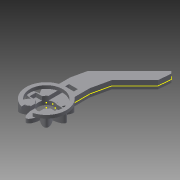
# Autodesk Inventor part: BrazoPinza2
Saved by Autodesk Inventor 2014 SP1 (Build 180222100, 222)
## iProperties
Created: 2013-11-10
Part Number: BrazoPinza2
Material: Genérico
Document SubType Name: Modeling
Designer: Gregorio
Density: 1 g/cm^3
Appearance: Valor por defecto
Author: Gregorio
Autodesk Inventor part; units mm, degrees
ref_plane "YZ Plane" through (0, 0, 0) normal (1, 0, 0) x (0, 1, 0)
ref_plane "XZ Plane" through (0, 0, 0) normal (0, 1, 0) x (-1, 0, 0)
ref_plane "XY Plane" through (0, 0, 0) normal (0, 0, 1) x (1, 0, 0)
sketch "Boceto1" plane through (0, 0, 0) normal (0, 0, 1) x (1, 0, 0)
  circle A0 centre (0, 0) radius 12.5
  circle A1 centre (0, 0) radius 4
  ellipse E0 centre (0, 4) end of major axis (0, 12.5) minor radius 3
  ellipse E1 centre (2.85, 2.8067) end of major axis (8.9175, 8.7595) minor radius 3
  ellipse E2 centre (4, 0) end of major axis (12.5, 0) minor radius 3
  ellipse E3 centre (2.85, -2.8067) end of major axis (8.8031, -8.8744) minor radius 3
  ellipse E4 centre (0, -4) end of major axis (0, -12.5) minor radius 3
  ellipse E5 centre (-2.85, -2.8067) end of major axis (-8.9175, -8.7595) minor radius 3
  ellipse E6 centre (-4, 0) end of major axis (-12.5, 0) minor radius 3
  ellipse E7 centre (-2.85, 2.8067) end of major axis (-8.8031, 8.8744) minor radius 3
  dimension "d1" = 8
  dimension "d4" = 3
  dimension "d5" = 3
  dimension "d6" = 3
  dimension "d7" = 3
  dimension "d8" = 3
  dimension "d9" = 3
  dimension "d10" = 3
  dimension "d11" = 3
  dimension "d0" = 25
  dimension "d12" = 2.85
  dimension "d14" = 2.85
  dimension "d15" = 2.85
  dimension "d16" = 2.85
  constraints: 2 coincident, 2 horizontal alignment, 2 vertical alignment, 1 centre point, 34 other
  measures "d0" diameter of A0
  measures "d12" horizontal distance of point (2.85, 2.807) point (0, 4)
  measures "d14" horizontal distance of point (-2.85, 2.807) point (0, 4)
  measures "d15" horizontal distance of point (0, -4) point (-2.85, -2.807)
  measures "d16" horizontal distance of point (2.85, -2.807) point (0, -4)
extrude "Extrusión1" add sketch "Boceto1" along normal blind 2 contours E2 E3 E6 E1 | E1 E2 E5 E0 | E3 E4 E7 E2 | E1 E6 A1 E5 E2 | E2 E7 A1 E6 E3 | E0 E1 E4 E7 | E0 E5 A1 E4 E1 | E4 E5 E0 E3 | E3 E0 A1 E7 E4 | E6 E3 E1 | E1 E3 A1 E6 | E5 A1 E0 E2 | E2 E0 E5 | E7 E4 E2 | E2 E4 A1 E7 | E6 A1 E1 E3 | E7 E0 E3 E6 | E7 E4 A1 E3 E0 | E0 E2 A1 E5 | E4 A1 E7 E1 | E1 E7 E4 | E5 E6 E1 E4 | E4 E1 A1 E0 E5 | E3 E5 A1 E0 | E0 E5 E3 | E7 A1 E2 E4 | E1 A1 E3 | E6 E5 A1 | A1 E3 E5 E6 | E0 A1 E2 | E5 E6 E0 A1 | E2 A1 E4 | E7 E6 A1 | A1 E4 E6 E7 | E6 E7 E1 A1 | E6 E7 E2 E5 | E6 E3 A1 E2 E7 | E3 A1 E6 E0 | E0 E6 E3 | E7 E1 A1 E4 | E5 E4 A1 | A1 E2 E4 E5 | E7 A1 E1 | E4 E5 E7 A1 | E5 E2 A1 E1 E6 | E4 E6 A1 E1 | E1 E6 E4 | E0 A1 E3 E5 | E0 E7 A1 | A1 E5 E7 E0 | E3 A1 E5 | E7 E0 E2 A1 | E1 E7 E5 E3 A1 | E5 E3 E0 E6 | E0 E6 E4 E2 A1 | E2 E0 E6 E4 A1 | E6 E4 E1 E7 | E6 E0 A1 E3 | E7 E5 E2 | E2 A1 E5 E7 | E6 A1 E0 | E3 E4 E6 A1 | A1 E4 E3 | A1 E1 E3 E4 | E4 E2 E7 E5 | A1 E7 E5 E3 E1 | E5 E7 A1 E2 | E1 A1 E4 E6 | E1 E0 A1 | A1 E6 E0 E1 | E4 A1 E6 | E0 E1 E3 A1 | A1 E3 E1 E7 E5 | E7 E5 E2 E0 | E1 E4 E5 E7 | E5 E7 E0 E3 | E0 E3 E4 E6 | E4 E6 E7 E2 | E2 E5 E6 E0 | E6 E0 E1 E4 | E3 E2 A1 | A1 E0 E2 E3 | E2 E3 E5 A1 | E5 A1 E7 | A1 E6 E4 E2 E0 | E3 E1 E6 E4 | E7 E2 E3 E5 | E3 E5 E6 E1 | E2 E1 A1 | A1 E7 E1 E2 | E1 E2 E4 A1 | A1 E4 E2 E0 E6 | E0 E6 E3 E1 | E7 E1 E2 E5 | E3 E6 E7 E1 | E1 E0 E5 E4 | E5 E4 E0 E7 | E0 E7 E4 E3 | E4 E3 E7 E6 | E7 E6 E3 E2 | E6 E5 E1 E0 | E2 E1 E6 E5 | E2 E0 E5 E3 | E5 E3 E1 E7 A1 | E2 E4 E5 E0 | E6 E1 E2 E4 | E3 E2 E6 E5 | E6 E5 E2 E1 | E1 E7 E4 E2 | E0 E2 E3 E6 | E4 E7 E0 E2 | E7 E6 E2 E1 | E3 E2 E7 E6 | E1 E5 E0 | E5 E0 E4 | E0 E4 E7 | E4 E7 E3 | E7 E3 E6 | E3 E6 E2 | E6 E1 E5 | E2 E6 E1 | E5 E0 E1 E3 | E1 E3 E4 E7 | E5 E4 E1 E0 | E2 E1 E5 E4 | E6 E2 E5 | E2 E5 E1 | E0 E7 E3 E2 | E4 E3 E0 E7 | E7 E2 E6 | E3 E7 E2 | E5 E1 E6 E2 E7 E3 E0 E4 | E1 E0 E4 E3 | E1 E4 E0 | E5 E1 E4 | E0 E3 E7 | E4 E0 E3
sketch "Boceto8" plane through (0, 0, 2) normal (0, 0, 1) x (1, 0, 0)
  ellipse E0 centre (0, -4) end of major axis (0, 4.5) minor radius 3 (-2.8365, -6.7677) -> (2.8299, -6.8216) ccw projected
  line L0 (-6, 0) -> (6, 0)
  line L1 (6, 0) -> (6, 30)
  line L2 (6, 30) -> (-6, 30)
  line L3 (-6, 30) -> (-6, 0)
  point P0 (-0.9996, -4.2411)
  point P1 (0.9996, -4.2411)
  point P2 (3.724, 2.2639)
  point P3 (2.3202, 3.6872)
  point P4 (-2.3223, 3.696)
  point P5 (-3.7155, 2.2614)
  dimension "d42" = 30
  constraints: 8 end point, 2 parallel, 1 horizontal, 1 perpendicular, 1 other
  measures "d42" distance of L1.end L0.end
extrude "Extrusión7" add sketch "Boceto8" along normal blind 3
sketch "Boceto3" plane through (0, 0, 2) normal (0, 0, 1) x (1, 0, 0)
  circle A0 centre (0, 0) radius 5
  dimension "d19" = 10
  constraints: 1 centre point
  measures "d19" diameter of A0
extrude "Extrusión2" cut sketch "Boceto3" along normal mid plane 10
sketch "Boceto23" plane through (0, 0, 2) normal (0, 0, 1) x (1, 0, 0)
  arc A0 (-5, 0) -> (5, 0) centre (0, 0) ccw projected
  line L0 (-5, 0) -> (-6, 0) projected
  line L1 (-6, 0) -> (-6, 8.7911) projected
  ellipse E0 centre (-2.85, 2.8067) end of major axis (3.1031, -3.261) minor radius 3 (-6, 8.7911) -> (-6.8377, 2.8279) ccw projected
  ellipse E1 centre (-4, 0) end of major axis (4.5, 0) minor radius 3 (-6.8377, 2.8279) -> (-6.8921, -2.821) ccw projected
  ellipse E2 centre (-2.85, -2.8067) end of major axis (3.2175, 3.1461) minor radius 3 (-6.8921, -2.821) -> (-2.8365, -6.7677) ccw projected
  ellipse E3 centre (0, -4) end of major axis (0, 4.5) minor radius 3 (-2.8365, -6.7677) -> (2.8299, -6.8216) ccw projected
  ellipse E4 centre (2.85, -2.8067) end of major axis (-3.1031, 3.261) minor radius 3 (2.8299, -6.8216) -> (6.8377, -2.8279) ccw projected
  ellipse E5 centre (4, 0) end of major axis (-4.5, 0) minor radius 3 (6.8377, -2.8279) -> (6.8921, 2.821) ccw projected
  ellipse E6 centre (2.85, 2.8067) end of major axis (-3.2175, -3.1461) minor radius 3 (6.8921, 2.821) -> (6, 8.6832) ccw projected
  line L2 (6, 8.6832) -> (6, 0) projected
  line L3 (6, 0) -> (5, 0) projected
  constraints: 7 other
extrude "Extrusión20" add sketch "Boceto23" along normal blind 3
sketch "Boceto14" plane through (0, 0, 5) normal (0, 0, 1) x (1, 0, 0)
  circle A0 centre (0, 0) radius 5 projected
  line L0 (-2.75, -17) -> (2.75, -17)
  line L1 (2.75, -17) -> (2.75, 17)
  line L2 (2.75, 17) -> (-2.75, 17)
  line L3 (-2.75, 17) -> (-2.75, -17)
  line L4 (-2.75, -17) -> (2.75, 17) construction
  line L5 (2.75, -17) -> (-2.75, 17) construction
  line L6 (-8.5, 2) -> (8.5, 2)
  line L7 (8.5, 2) -> (8.5, -2)
  line L8 (8.5, -2) -> (-8.5, -2)
  line L9 (-8.5, -2) -> (-8.5, 2)
  line L10 (-8.5, 2) -> (8.5, -2) construction
  line L11 (8.5, 2) -> (-8.5, -2) construction
  dimension "d45" = 5.5
  dimension "d46" = 34
  dimension "d47" = 17
  dimension "d48" = 4
  constraints: 24 end point, 4 midpoint, 4 parallel, 2 horizontal, 2 perpendicular
  measures "d45" distance of L2.end L1.end
  measures "d46" distance of L1.end L0.end
  measures "d47" distance of L7.end L8.end
  measures "d48" distance of L6.end L7.end
extrude "Extrusión12" cut sketch "Boceto14" against normal blind 2.5 contours A0 L8 L1 L6 | A0 L6 L7 L8 | A0 L3 L2 L1 | L1 L8 L3 L6 | L1 L0 L3 A0 | L3 L8 A0 L6 | A0 L8 L9 L6
sketch "Boceto24" plane through (0, 0, 5) normal (0, 0, 1) x (1, 0, 0)
  line L0 (6, 30) -> (1, 35)
  line L1 (1, 35) -> (22.2132, 56.2132)
  line L2 (22.2132, 56.2132) -> (27.2132, 51.2132)
  line L3 (27.2132, 51.2132) -> (6, 30)
  line L4 (6, 30) -> (-6, 30) projected
  dimension "d80" = 30
  dimension "d81" = 5
  dimension "d92" = 45
  constraints: 8 end point, 2 parallel, 1 perpendicular
  measures "d80" distance of L0.end L1.end
  measures "d81" horizontal distance of L0.start L0.end
  measures "d92" angle of L4 L0
extrude "Extrusión21" add sketch "Boceto24" against normal blind 3
sketch "Boceto26" plane through (1, 35, 5) normal (-0.7071068, -0.7071068, 0) x (-0.7071068, 0.7071068, 0)
  line L0 (0, 0) -> (-7.0711, 0) projected
  line L1 (0, 0) -> (0, 3) projected
  line L2 (-7.0711, 3) -> (0, 3) projected
  line L3 (-7.0711, 3) -> (-7.0711, 0) projected
  point P0 (-24.0416, 5)
extrude "Extrusión23" add sketch "Boceto26" along normal up to next
sketch "Boceto27" plane through (0, 0, 5) normal (0, 0, 1) x (1, 0, 0)
  line L0 (-4, 30) -> (-5.9524, 21.2143)
  line L1 (-5.9524, 21.2143) -> (-13.0465, 22.7908)
  line L2 (-13.0465, 22.7908) -> (-11.0941, 31.5765)
  line L3 (-11.0941, 31.5765) -> (-4, 30)
  dimension "d94" = 9
  constraints: 8 end point, 2 parallel, 1 perpendicular
  measures "d94" distance of L1.end L2.end
extrude "Extrusión24" cut sketch "Boceto27" against normal blind 3
sketch "Boceto28" plane through (0, 0, 5) normal (0, 0, 1) x (1, 0, 0)
  line L0 (-4, 30) -> (-5.9524, 21.2143) projected
  line L1 (6, 8.6832) -> (6, 30) projected
  line L2 (6, 30) -> (27.2132, 51.2132) projected
  line L3 (6, 21.25) -> (8.5, 32.5)
  line L4 (8.5, 32.5) -> (5.0588, 33.2647)
  line L5 (5.0588, 33.2647) -> (2.5588, 22.0147)
  line L6 (2.5588, 22.0147) -> (6, 21.25)
  point P0 (-6, 21)
  dimension "d95" = 2.5
  constraints: 8 end point, 3 parallel, 2 point on line, 1 perpendicular
  measures "d95" horizontal distance of L3.end L1.end
extrude "Extrusión25" add sketch "Boceto28" against normal blind 3 contours L1 L2 L3
chamfer "Chaflán5" distance 5 angle 50 1 edges at (27.2132, 51.2132, 3.5) measured on face at (26.8597, 51.5668, 3.5)
sketch "Boceto29" plane through (0, 0, 5) normal (0, 0, 1) x (1, 0, 0)
  arc A0 (4.5826, 2) -> (2.75, 4.1758) centre (0, 0) ccw projected
  circle A1 centre (0, 0) radius 12.6015
  circle A2 centre (0, 0) radius 10.2854
  constraints: 2 centre point, 2 coincident
extrude "Extrusión26" add sketch "Boceto29" along normal blind 2
sketch "Boceto30" plane through (0, 0, 7) normal (0, 0, 1) x (1, 0, 0)
  circle A0 centre (0, 0) radius 10.2854 projected
  line L0 (-3.5, 0) -> (3.5, 0)
  line L1 (3.5, 0) -> (3.5, -17)
  line L2 (3.5, -17) -> (-3.5, -17)
  line L3 (-3.5, -17) -> (-3.5, 0)
  point P0 (0, 0)
  dimension "d101" = 7
  constraints: 8 end point, 2 parallel, 1 coincident, 1 horizontal, 1 midpoint, 1 perpendicular
  measures "d101" distance of L1.end L2.end
extrude "Extrusión27" cut sketch "Boceto30" against normal blind 2 contours L3 L0 L1 A0 | A0 L1 L2 L3 picked at (-0.3959, -3.4055)
sketch "Boceto31" plane through (0, 0, 2) normal (0, 0, -1) x (-1, 0, 0)
  line L0 (-22.9997, 46.9997) -> (-23.6777, 54.7487) projected
  line L1 (-22.9997, 46.9997) -> (-8.5, 32.5) projected
  line L2 (-8.5, 32.5) -> (-6, 21.25) projected
  line L3 (-6, 8.6832) -> (-6, 21.25) projected
  ellipse E0 centre (-2.85, 2.8067) end of major axis (3.2175, -3.1461) minor radius 3 (-2.8365, 6.7677) -> (-6, 8.6832) ccw projected
  ellipse E1 centre (0, 4) end of major axis (0, -4.5) minor radius 3 (2.8299, 6.8216) -> (-2.8365, 6.7677) ccw projected
  ellipse E2 centre (2.85, 2.8067) end of major axis (-3.1031, -3.261) minor radius 3 (6, 8.7911) -> (2.8299, 6.8216) ccw projected
  line L4 (6, 21.2249) -> (6, 8.7911) projected
  line L5 (6, 21.2249) -> (5.9524, 21.2143) projected
  line L6 (5.9524, 21.2143) -> (4, 30) projected
  line L7 (-22.2132, 56.2132) -> (4, 30) projected
  line L8 (-22.2132, 56.2132) -> (-23.6777, 54.7487) projected
  point P0 (0, 0)
  constraints: 3 other
sketch "Boceto32" plane through (0, 0, 2) normal (0, 0, -1) x (-1, 0, 0)
  line L0 (-22.9997, 46.9997) -> (-23.6777, 54.7487) projected
  line L1 (-22.9997, 46.9997) -> (-8.5, 32.5) projected
  line L2 (-8.5, 32.5) -> (-6, 21.25) projected
  line L3 (-6, 8.6832) -> (-6, 21.25) projected
  ellipse E0 centre (-2.85, 2.8067) end of major axis (3.2175, -3.1461) minor radius 3 (-2.8365, 6.7677) -> (-6, 8.6832) ccw projected
  ellipse E1 centre (0, 4) end of major axis (0, -4.5) minor radius 3 (2.8299, 6.8216) -> (-2.8365, 6.7677) ccw projected
  ellipse E2 centre (2.85, 2.8067) end of major axis (-3.1031, -3.261) minor radius 3 (6, 8.7911) -> (2.8299, 6.8216) ccw projected
  line L4 (6, 21.2249) -> (6, 8.7911) projected
  line L5 (6, 21.2249) -> (5.9524, 21.2143) projected
  line L6 (5.9524, 21.2143) -> (4, 30) projected
  line L7 (-22.2132, 56.2132) -> (4, 30) projected
  line L8 (-22.2132, 56.2132) -> (-23.6777, 54.7487) projected
  point P0 (0, 0)
  constraints: 3 other
extrude "Extrusión28" add sketch "Boceto31" along normal blind 2
